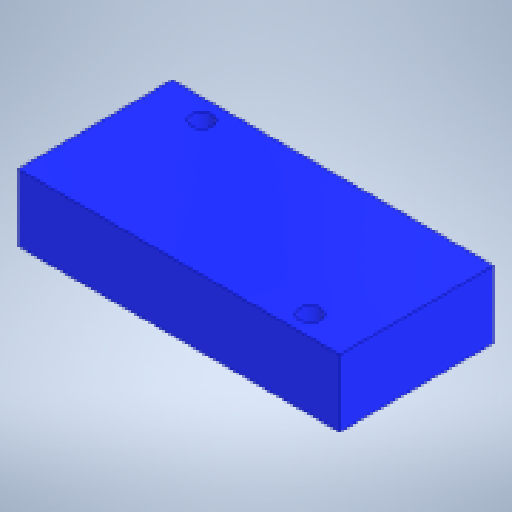
# Autodesk Inventor part: стабилизатор
Saved by Autodesk Inventor 2023.1 (Build 271208000, 208)
## iProperties
Created: 2025-01-21
Part Number: стабилизатор
Material: Типовые
Document SubType Name: Modeling
Designer: DELL
Density: 1 g/cm^3
Appearance: Синий — малярная краска — глянцевая
Author: DELL
Autodesk Inventor part; units mm, degrees
ref_plane "YZ Plane" through (0, 0, 0) normal (1, 0, 0) x (0, 1, 0)
ref_plane "XZ Plane" through (0, 0, 0) normal (0, 1, 0) x (-1, 0, 0)
ref_plane "XY Plane" through (0, 0, 0) normal (0, 0, 1) x (1, 0, 0)
sketch "Эскиз1" plane through (0, 0, 0) normal (0, 1, 0) x (-1, 0, 0)
  line L0 (24, -11.5) -> (-24, -11.5)
  line L1 (-24, -11.5) -> (-24, 11.5)
  line L2 (-24, 11.5) -> (24, 11.5)
  line L3 (24, 11.5) -> (24, -11.5)
  line L4 (24, -11.5) -> (-24, 11.5) construction
  line L5 (-24, -11.5) -> (24, 11.5) construction
  point P0 (0, 0)
  dimension "d0" = 48
  dimension "d1" = 23
  constraints: 12 end point, 2 midpoint, 2 parallel, 1 horizontal, 1 perpendicular
  measures "d0" distance of L1.end L2.end
  measures "d1" distance of L0.end L1.end
extrude "Выдавливание1" add sketch "Эскиз1" along normal blind 10
sketch "Эскиз2" plane through (0, 10, 0) normal (0, 1, 0) x (1, 0, 0)
  circle A0 centre (16.58, -8.5) radius 1.575
  circle A1 centre (-16.58, 8.5) radius 1.575
  line L0 (24, -11.5) -> (24, 11.5) projected
  line L1 (-24, -11.5) -> (24, -11.5) projected
  line L2 (24, 11.5) -> (-24, 11.5) projected
  line L3 (-24, 11.5) -> (-24, -11.5) projected
  point P0 (0, 0)
  dimension "d4" = 3.15
  dimension "d5" = 3.15
  dimension "d6" = 40.58
  dimension "d7" = 20
  dimension "d8" = 20
  dimension "d9" = 40.58
  constraints: 2 centre point
  measures "d4" diameter of A0
  measures "d5" diameter of A1
  measures "d6" distance from line of L0 A1.centre
  measures "d7" distance from line of A1.centre L1
  measures "d8" distance from line of A0.centre L2
  measures "d9" distance from line of L3 A0.centre
extrude "Выдавливание2" cut sketch "Эскиз2" against normal blind 10 contours A0 | A1
